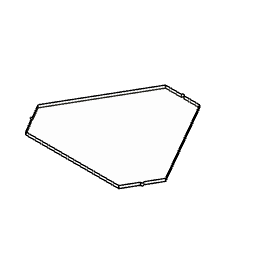
Zusammenbau v36 (Autodesk Fusion 360 archive; units mm, degrees)
design "Diffusor_Panel"
Autodesk Fusion 360 part; units mm, degrees
note: some values were not read from the file. Set by a fixed rule: the direction of a hole.
(part 1 of 2)
sketch "Skizze1" plane through (0, 0, 0) normal (0, 0, 1) x (1, 0, 0)
  line L0 (-53.4049, 0) -> (53.4049, 0)
  line L1 (53.4049, 0) -> (73.0348, 34)
  line L2 (73.0348, 34) -> (19.6299, 126.5)
  line L3 (19.6299, 126.5) -> (-19.6299, 126.5)
  line L4 (-19.6299, 126.5) -> (-73.0348, 34)
  line L5 (-73.0348, 34) -> (-53.4049, 0)
  line L6 (0, 0) -> (0, 126.5)
  line L7 (-63.2199, 17) -> (46.3324, 80.25)
  line L8 (63.2199, 17) -> (-46.3324, 80.25)
  circle A0 centre (0, 126.5) radius 1.4
  circle A1 centre (-63.2199, 17) radius 1.4
  circle A2 centre (63.2199, 17) radius 1.4
  point P0 (0, 53.5)
  dimension "d1" = 53.5
  dimension "d2" = 73
  dimension "d3" = 39.2598
  dimension "d4" = 106.8098
  dimension "d11" = 2.8
  dimension "d13" = 360
  constraint horizontal L0
  constraint parallel L0 L3
  constraint parallel L1 L4
  constraint equal L1 L3
  constraint equal L1 L5
  constraint equal L2 L4
  constraint equal L0 L2
  constraint coincident L6.start L0
  constraint coincident L6.start origin
  constraint coincident L3 L6.end
  constraint perpendicular L3 L6
  constraint symmetric L2 L4 L6
  constraint symmetric L1 L5 L6
  constraint midpoint L5 L7.start
  constraint midpoint L2 L7.end
  constraint midpoint L1 L8.start
  constraint midpoint L4 L8.end
  constraint coincident L7 P0
  constraint coincident L6 P0
  constraint coincident L6.end A0.centre
  measures "d1" distance of L0 P0
  measures "d2" distance of L3 P0
  measures "d3" distance of L2.end L3.end
  measures "d4" distance of L0.start L0.end
  measures "d11" diameter of A0
extrude "Extrusion1" add sketch "Skizze1" along normal blind 3
sketch "Skizze2" plane through (0, 0, 3) normal (0, 0, 1) x (-1, 0, 0)
  arc A0 (-62.5199, -15.7876) -> (-63.9199, -18.2124) centre (-63.2199, -17) ccw
  line L0 (-63.9199, -18.2124) -> (-73.0348, -34)
  line L1 (-73.0348, -34) -> (-19.6299, -126.5)
  line L2 (-19.6299, -126.5) -> (-1.4, -126.5)
  arc A1 (-1.4, -126.5) -> (1.4, -126.5) centre (0, -126.5) ccw
  line L3 (1.4, -126.5) -> (19.6299, -126.5)
  line L4 (19.6299, -126.5) -> (73.0348, -34)
  line L5 (73.0348, -34) -> (63.9199, -18.2124)
  arc A2 (63.9199, -18.2124) -> (62.5199, -15.7876) centre (63.2199, -17) ccw
  line L6 (62.5199, -15.7876) -> (53.4049, 0)
  line L7 (53.4049, 0) -> (-53.4049, 0)
  line L8 (-53.4049, 0) -> (-62.5199, -15.7876)
equation "d6 = 0deg 0'"
equation "d10 = 0deg 0'"
equation "d13 = 360deg 0'"

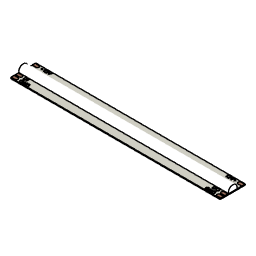
design "FCOB"
Autodesk Fusion 360 part; units mm, degrees
sketch "Skizze1" plane through (0, 0, 0) normal (1, 0, 0) x (0, 1, 0)
  line L0 (0, 0) -> (12, 0)
  line L1 (12, 0) -> (12, 0.4)
  line L2 (12, 0.4) -> (0, 0.4)
  line L3 (0, 0.4) -> (0, 0)
  arc A0 (8, 0.4) -> (4, 0.4) centre (6, 1.0093) ccw
  line L4 (6, 0.4) -> (6, 0)
  point P0 (6, 3.1)
  dimension "d1" = 0.4
  dimension "d2" = 12
  dimension "d3" = 3.1
  dimension "d4" = 4
  constraint horizontal L0
  constraint vertical L1
  constraint horizontal L2
  constraint vertical L3
  constraint coincident L0.start L3.end
  constraint coincident L2 A0.start
  constraint coincident L2 A0.end
  constraint midpoint L2 L4.start
  constraint midpoint L0 L4.end
  constraint coincident A0.centre L4
  constraint midpoint A0 P0
  measures "d1" distance of L0.start L2.end
  measures "d2" distance of L1.end L2.end
  measures "d3" distance of L0 P0
  measures "d4" distance of A0.end A0.start
extrude "Extrusion1" add sketch "Skizze1" along normal blind 100 contours L0 L2 L3 L4 | L0 L1 L2 L4 makes body 1
extrude "Extrusion2" add sketch "Skizze1" along normal up to surface (100 mm away) separate body contours L2 A0 makes body 2
sketch "Skizze2" plane through (0, 0, 0.4) normal (0, 0, 1) x (-1, 0, 0)
  line L0 (0, -12) -> (0, 0)
  line L1 (0, 0) -> (-100, 0)
  line L2 (-100, 0) -> (-100, -12)
  line L3 (-100, -12) -> (0, -12)
  line L4 (0, -0.25) -> (0, -1.75)
  line L5 (-1.75, -1.75) -> (0, -1.75)
  line L6 (0, -0.25) -> (-1.75, -0.25)
  arc A0 (-1.75, -0.25) -> (-1.75, -1.75) centre (-1.75, -1) ccw
  line L7 (0, -1) -> (-2.5, -1) construction
  dimension "d11" = 1.5
  dimension "d13" = 2.5
  dimension "d14" = 0.25
  constraint coincident L0 L4.start
  constraint coincident L0 L4.end
  constraint perpendicular L4 L5
  constraint perpendicular L4 L6
  constraint tangent L6 A0
  constraint tangent L5 A0
  constraint midpoint L4 L7.start
  constraint midpoint A0 L7.end
  measures "d11" distance of L4.start L4.end
  measures "d13" distance of L7.start L7.end
  measures "d14" distance of L1 L6
extrude "Extrusion3" add sketch "Skizze2" along normal blind 0.035 contours L0 L4 L5 L6 A0 bodies 1
pattern_linear "R-Anordnung1" count 2 spacing 2 along (0, 1, 0) of "Extrusion3"
pattern_linear "R-Anordnung2" count 2 spacing 10 along (0, 1, 0) of "Extrusion3"
ref_plane "Arbeitsebene1" through (50, 6, 0.2175) normal (-1, 0, 0) x (0, -1, 0)
mirror "Spiegeln1" about plane through (50, 6, 0.2175) normal (-1, 0, 0) of "Extrusion3", "R-Anordnung1", "R-Anordnung2"
sketch "Skizze3" plane through (0, 0, 0.4) normal (0, 0, 1) x (-1, 0, 0)
  line L0 (-100, -10.25) -> (-98.25, -10.25)
  arc A0 (-98.25, -11.75) -> (-98.25, -10.25) centre (-98.25, -11) ccw
  line L1 (-98.25, -11.75) -> (-100, -11.75)
  line L2 (-100, -11.75) -> (-100, -12)
  line L3 (-100, -12) -> (0, -12)
  line L4 (0, -12) -> (0, -11.75)
  line L5 (0, -11.75) -> (-1.75, -11.75)
  arc A1 (-1.75, -10.25) -> (-1.75, -11.75) centre (-1.75, -11) ccw
  line L6 (-1.75, -10.25) -> (0, -10.25)
  line L7 (0, -10.25) -> (0, -3.75)
  line L8 (0, -3.75) -> (-1.75, -3.75)
  arc A2 (-1.75, -2.25) -> (-1.75, -3.75) centre (-1.75, -3) ccw
  line L9 (-1.75, -2.25) -> (0, -2.25)
  line L10 (0, -2.25) -> (0, -1.75)
  line L11 (0, -1.75) -> (-1.75, -1.75)
  arc A3 (-1.75, -0.25) -> (-1.75, -1.75) centre (-1.75, -1) ccw
  line L12 (-1.75, -0.25) -> (0, -0.25)
  line L13 (0, -0.25) -> (0, 0)
  line L14 (0, 0) -> (-100, 0)
  line L15 (-100, 0) -> (-100, -0.25)
  line L16 (-100, -0.25) -> (-98.25, -0.25)
  arc A4 (-98.25, -1.75) -> (-98.25, -0.25) centre (-98.25, -1) ccw
  line L17 (-98.25, -1.75) -> (-100, -1.75)
  line L18 (-100, -1.75) -> (-100, -2.25)
  line L19 (-100, -2.25) -> (-98.25, -2.25)
  arc A5 (-98.25, -3.75) -> (-98.25, -2.25) centre (-98.25, -3) ccw
  line L20 (-98.25, -3.75) -> (-100, -3.75)
  line L21 (-100, -3.75) -> (-100, -10.25)
  line L22 (-4.252, -0.8383) -> (-4.252, -1.0143)
  line L23 (-4.252, -1.0143) -> (-4.8874, -1.0153)
  line L24 (-4.8874, -1.0153) -> (-4.8874, -0.4587)
  spline S0 degree 2 poles (-4.8874, -0.4587) (-4.7411, -0.3421) (-4.5856, -0.2833) knots 0 0 0 1 1 1
  spline S1 degree 2 poles (-4.5856, -0.2833) (-4.4301, -0.2244) (-4.2664, -0.2244) knots 0 0 0 1 1 1
  spline S2 degree 2 poles (-4.2664, -0.2244) (-4.0454, -0.2244) (-3.8648, -0.3191) knots 0 0 0 1 1 1
  spline S3 degree 2 poles (-3.8648, -0.3191) (-3.6842, -0.4137) (-3.5921, -0.5928) knots 0 0 0 1 1 1
  spline S4 degree 2 poles (-3.5921, -0.5928) (-3.5, -0.7718) (-3.5, -0.9928) knots 0 0 0 1 1 1
  spline S5 degree 2 poles (-3.5, -0.9928) (-3.5, -1.2118) (-3.5916, -1.4016) knots 0 0 0 1 1 1
  spline S6 degree 2 poles (-3.5916, -1.4016) (-3.6832, -1.5914) (-3.855, -1.6835) knots 0 0 0 1 1 1
  spline S7 degree 2 poles (-3.855, -1.6835) (-4.0269, -1.7756) (-4.251, -1.7756) knots 0 0 0 1 1 1
  spline S8 degree 2 poles (-4.251, -1.7756) (-4.4137, -1.7756) (-4.5452, -1.7229) knots 0 0 0 1 1 1
  spline S9 degree 2 poles (-4.5452, -1.7229) (-4.6767, -1.6702) (-4.7514, -1.5761) knots 0 0 0 1 1 1
  spline S10 degree 2 poles (-4.7514, -1.5761) (-4.8261, -1.4819) (-4.8649, -1.3305) knots 0 0 0 1 1 1
  line L25 (-4.8649, -1.3305) -> (-4.6859, -1.2814)
  spline S11 degree 2 poles (-4.6859, -1.2814) (-4.6521, -1.396) (-4.602, -1.4615) knots 0 0 0 1 1 1
  spline S12 degree 2 poles (-4.602, -1.4615) (-4.5518, -1.5269) (-4.4587, -1.5663) knots 0 0 0 1 1 1
  spline S13 degree 2 poles (-4.4587, -1.5663) (-4.3656, -1.6057) (-4.252, -1.6057) knots 0 0 0 1 1 1
  spline S14 degree 2 poles (-4.252, -1.6057) (-4.116, -1.6057) (-4.0167, -1.5643) knots 0 0 0 1 1 1
  spline S15 degree 2 poles (-4.0167, -1.5643) (-3.9175, -1.5229) (-3.8566, -1.4553) knots 0 0 0 1 1 1
  spline S16 degree 2 poles (-3.8566, -1.4553) (-3.7957, -1.3878) (-3.7619, -1.307) knots 0 0 0 1 1 1
  spline S17 degree 2 poles (-3.7619, -1.307) (-3.7046, -1.1678) (-3.7046, -1.0051) knots 0 0 0 1 1 1
  spline S18 degree 2 poles (-3.7046, -1.0051) (-3.7046, -0.8046) (-3.7737, -0.6695) knots 0 0 0 1 1 1
  spline S19 degree 2 poles (-3.7737, -0.6695) (-3.8428, -0.5344) (-3.9748, -0.469) knots 0 0 0 1 1 1
  spline S20 degree 2 poles (-3.9748, -0.469) (-4.1068, -0.4035) (-4.2551, -0.4035) knots 0 0 0 1 1 1
  spline S21 degree 2 poles (-4.2551, -0.4035) (-4.384, -0.4035) (-4.5068, -0.4531) knots 0 0 0 1 1 1
  spline S22 degree 2 poles (-4.5068, -0.4531) (-4.6296, -0.5027) (-4.693, -0.559) knots 0 0 0 1 1 1
  line L26 (-4.693, -0.559) -> (-4.693, -0.8383)
  line L27 (-4.693, -0.8383) -> (-4.252, -0.8383)
  line L28 (-5.178, -0.25) -> (-5.178, -1.75)
  line L29 (-5.178, -1.75) -> (-5.3817, -1.75)
  line L30 (-5.3817, -1.75) -> (-6.1695, -0.5723)
  line L31 (-6.1695, -0.5723) -> (-6.1695, -1.75)
  line L32 (-6.1695, -1.75) -> (-6.3598, -1.75)
  line L33 (-6.3598, -1.75) -> (-6.3598, -0.25)
  line L34 (-6.3598, -0.25) -> (-6.1562, -0.25)
  line L35 (-6.1562, -0.25) -> (-5.3683, -1.4287)
  line L36 (-5.3683, -1.4287) -> (-5.3683, -0.25)
  line L37 (-5.3683, -0.25) -> (-5.178, -0.25)
  line L38 (-6.6934, -0.25) -> (-6.6934, -1.75)
  line L39 (-6.6934, -1.75) -> (-7.2101, -1.75)
  spline S23 degree 2 poles (-7.2101, -1.75) (-7.3851, -1.75) (-7.4771, -1.7285) knots 0 0 0 1 1 1
  spline S24 degree 2 poles (-7.4771, -1.7285) (-7.6061, -1.6988) (-7.6971, -1.6211) knots 0 0 0 1 1 1
  spline S25 degree 2 poles (-7.6971, -1.6211) (-7.8158, -1.5208) (-7.8747, -1.3648) knots 0 0 0 1 1 1
  spline S26 degree 2 poles (-7.8747, -1.3648) (-7.9335, -1.2087) (-7.9335, -1.0082) knots 0 0 0 1 1 1
  spline S27 degree 2 poles (-7.9335, -1.0082) (-7.9335, -0.8373) (-7.8936, -0.7053) knots 0 0 0 1 1 1
  spline S28 degree 2 poles (-7.8936, -0.7053) (-7.8537, -0.5733) (-7.7913, -0.4869) knots 0 0 0 1 1 1
  spline S29 degree 2 poles (-7.7913, -0.4869) (-7.7289, -0.4004) (-7.6547, -0.3508) knots 0 0 0 1 1 1
  spline S30 degree 2 poles (-7.6547, -0.3508) (-7.5805, -0.3012) (-7.4756, -0.2756) knots 0 0 0 1 1 1
  spline S31 degree 2 poles (-7.4756, -0.2756) (-7.3707, -0.25) (-7.2347, -0.25) knots 0 0 0 1 1 1
  line L40 (-7.2347, -0.25) -> (-6.6934, -0.25)
  line L41 (-6.8919, -0.427) -> (-7.2121, -0.427)
  spline S32 degree 2 poles (-7.2121, -0.427) (-7.3605, -0.427) (-7.4449, -0.4546) knots 0 0 0 1 1 1
  spline S33 degree 2 poles (-7.4449, -0.4546) (-7.5293, -0.4823) (-7.5795, -0.5324) knots 0 0 0 1 1 1
  spline S34 degree 2 poles (-7.5795, -0.5324) (-7.6501, -0.603) (-7.6895, -0.7222) knots 0 0 0 1 1 1
  spline S35 degree 2 poles (-7.6895, -0.7222) (-7.7289, -0.8414) (-7.7289, -1.0113) knots 0 0 0 1 1 1
  spline S36 degree 2 poles (-7.7289, -1.0113) (-7.7289, -1.2466) (-7.6516, -1.373) knots 0 0 0 1 1 1
  spline S37 degree 2 poles (-7.6516, -1.373) (-7.5744, -1.4993) (-7.4638, -1.5423) knots 0 0 0 1 1 1
  spline S38 degree 2 poles (-7.4638, -1.5423) (-7.384, -1.573) (-7.207, -1.573) knots 0 0 0 1 1 1
  line L42 (-7.207, -1.573) -> (-6.8919, -1.573)
  line L43 (-6.8919, -1.573) -> (-6.8919, -0.427)
  line L44 (-3.5, -2.25) -> (-3.5, -3.75)
  line L45 (-3.5, -3.75) -> (-4.0167, -3.75)
  spline S39 degree 2 poles (-4.0167, -3.75) (-4.1917, -3.75) (-4.2838, -3.7285) knots 0 0 0 1 1 1
  spline S40 degree 2 poles (-4.2838, -3.7285) (-4.4127, -3.6988) (-4.5038, -3.6211) knots 0 0 0 1 1 1
  spline S41 degree 2 poles (-4.5038, -3.6211) (-4.6224, -3.5208) (-4.6813, -3.3648) knots 0 0 0 1 1 1
  spline S42 degree 2 poles (-4.6813, -3.3648) (-4.7401, -3.2087) (-4.7401, -3.0082) knots 0 0 0 1 1 1
  spline S43 degree 2 poles (-4.7401, -3.0082) (-4.7401, -2.8373) (-4.7002, -2.7053) knots 0 0 0 1 1 1
  spline S44 degree 2 poles (-4.7002, -2.7053) (-4.6603, -2.5733) (-4.5979, -2.4869) knots 0 0 0 1 1 1
  spline S45 degree 2 poles (-4.5979, -2.4869) (-4.5355, -2.4004) (-4.4613, -2.3508) knots 0 0 0 1 1 1
  spline S46 degree 2 poles (-4.4613, -2.3508) (-4.3871, -2.3012) (-4.2822, -2.2756) knots 0 0 0 1 1 1
  spline S47 degree 2 poles (-4.2822, -2.2756) (-4.1774, -2.25) (-4.0413, -2.25) knots 0 0 0 1 1 1
  line L46 (-4.0413, -2.25) -> (-3.5, -2.25)
  line L47 (-3.6985, -2.427) -> (-4.0188, -2.427)
  spline S48 degree 2 poles (-4.0188, -2.427) (-4.1671, -2.427) (-4.2515, -2.4546) knots 0 0 0 1 1 1
  spline S49 degree 2 poles (-4.2515, -2.4546) (-4.3359, -2.4823) (-4.3861, -2.5324) knots 0 0 0 1 1 1
  spline S50 degree 2 poles (-4.3861, -2.5324) (-4.4567, -2.603) (-4.4961, -2.7222) knots 0 0 0 1 1 1
  spline S51 degree 2 poles (-4.4961, -2.7222) (-4.5355, -2.8414) (-4.5355, -3.0113) knots 0 0 0 1 1 1
  spline S52 degree 2 poles (-4.5355, -3.0113) (-4.5355, -3.2466) (-4.4582, -3.373) knots 0 0 0 1 1 1
  spline S53 degree 2 poles (-4.4582, -3.373) (-4.381, -3.4993) (-4.2705, -3.5423) knots 0 0 0 1 1 1
  spline S54 degree 2 poles (-4.2705, -3.5423) (-4.1907, -3.573) (-4.0136, -3.573) knots 0 0 0 1 1 1
  line L48 (-4.0136, -3.573) -> (-3.6985, -3.573)
  line L49 (-3.6985, -3.573) -> (-3.6985, -2.427)
  line L50 (-5.0471, -2.25) -> (-5.0471, -3.75)
  line L51 (-5.0471, -3.75) -> (-5.2456, -3.75)
  line L52 (-5.2456, -3.75) -> (-5.2456, -2.25)
  line L53 (-5.2456, -2.25) -> (-5.0471, -2.25)
  line L54 (-3.9083, -10.4925) -> (-3.9083, -10.9038)
  line L55 (-3.9083, -10.9038) -> (-3.5, -10.9038)
  line L56 (-3.5, -10.9038) -> (-3.5, -11.0757)
  line L57 (-3.5, -11.0757) -> (-3.9083, -11.0757)
  line L58 (-3.9083, -11.0757) -> (-3.9083, -11.484)
  line L59 (-3.9083, -11.484) -> (-4.0822, -11.484)
  line L60 (-4.0822, -11.484) -> (-4.0822, -11.0757)
  line L61 (-4.0822, -11.0757) -> (-4.4905, -11.0757)
  line L62 (-4.4905, -11.0757) -> (-4.4905, -10.9038)
  line L63 (-4.4905, -10.9038) -> (-4.0822, -10.9038)
  line L64 (-4.0822, -10.9038) -> (-4.0822, -10.4925)
  line L65 (-4.0822, -10.4925) -> (-3.9083, -10.4925)
  line L66 (-5.3878, -10.25) -> (-5.2036, -10.25)
  line L67 (-5.2036, -10.25) -> (-5.2036, -11.4236)
  spline S55 degree 2 poles (-5.2036, -11.4236) (-5.1371, -11.3602) (-5.0292, -11.2967) knots 0 0 0 1 1 1
  spline S56 degree 2 poles (-5.0292, -11.2967) (-4.9212, -11.2333) (-4.8353, -11.2016) knots 0 0 0 1 1 1
  line L68 (-4.8353, -11.2016) -> (-4.8353, -11.3796)
  spline S57 degree 2 poles (-4.8353, -11.3796) (-4.9898, -11.4523) (-5.1054, -11.5556) knots 0 0 0 1 1 1
  spline S58 degree 2 poles (-5.1054, -11.5556) (-5.221, -11.6589) (-5.2691, -11.7561) knots 0 0 0 1 1 1
  line L69 (-5.2691, -11.7561) -> (-5.3878, -11.7561)
  line L70 (-5.3878, -11.7561) -> (-5.3878, -10.25)
  line L71 (-6.8274, -10.427) -> (-6.8274, -10.25)
  line L72 (-6.8274, -10.25) -> (-5.8359, -10.25)
  spline S59 degree 2 poles (-5.8359, -10.25) (-5.8339, -10.3165) (-5.8574, -10.3779) knots 0 0 0 1 1 1
  spline S60 degree 2 poles (-5.8574, -10.3779) (-5.8953, -10.4792) (-5.9787, -10.5774) knots 0 0 0 1 1 1
  spline S61 degree 2 poles (-5.9787, -10.5774) (-6.0621, -10.6756) (-6.2196, -10.8046) knots 0 0 0 1 1 1
  spline S62 degree 2 poles (-6.2196, -10.8046) (-6.4642, -11.0051) (-6.5501, -11.1223) knots 0 0 0 1 1 1
  spline S63 degree 2 poles (-6.5501, -11.1223) (-6.6361, -11.2394) (-6.6361, -11.3438) knots 0 0 0 1 1 1
  spline S64 degree 2 poles (-6.6361, -11.3438) (-6.6361, -11.4533) (-6.5578, -11.5285) knots 0 0 0 1 1 1
  spline S65 degree 2 poles (-6.5578, -11.5285) (-6.4795, -11.6037) (-6.3537, -11.6037) knots 0 0 0 1 1 1
  spline S66 degree 2 poles (-6.3537, -11.6037) (-6.2207, -11.6037) (-6.1409, -11.5239) knots 0 0 0 1 1 1
  spline S67 degree 2 poles (-6.1409, -11.5239) (-6.0611, -11.4441) (-6.06, -11.3029) knots 0 0 0 1 1 1
  line L73 (-6.06, -11.3029) -> (-5.8707, -11.3223)
  spline S68 degree 2 poles (-5.8707, -11.3223) (-5.8902, -11.5341) (-6.0171, -11.6451) knots 0 0 0 1 1 1
  spline S69 degree 2 poles (-6.0171, -11.6451) (-6.1439, -11.7561) (-6.3578, -11.7561) knots 0 0 0 1 1 1
  spline S70 degree 2 poles (-6.3578, -11.7561) (-6.5737, -11.7561) (-6.6995, -11.6364) knots 0 0 0 1 1 1
  spline S71 degree 2 poles (-6.6995, -11.6364) (-6.8254, -11.5167) (-6.8254, -11.3397) knots 0 0 0 1 1 1
  spline S72 degree 2 poles (-6.8254, -11.3397) (-6.8254, -11.2497) (-6.7885, -11.1627) knots 0 0 0 1 1 1
  spline S73 degree 2 poles (-6.7885, -11.1627) (-6.7517, -11.0757) (-6.6663, -10.9795) knots 0 0 0 1 1 1
  spline S74 degree 2 poles (-6.6663, -10.9795) (-6.5808, -10.8834) (-6.3823, -10.7156) knots 0 0 0 1 1 1
  spline S75 degree 2 poles (-6.3823, -10.7156) (-6.2166, -10.5764) (-6.1695, -10.5268) knots 0 0 0 1 1 1
  spline S76 degree 2 poles (-6.1695, -10.5268) (-6.1224, -10.4771) (-6.0917, -10.427) knots 0 0 0 1 1 1
  line L74 (-6.0917, -10.427) -> (-6.8274, -10.427)
  line L75 (-7.5283, -10.25) -> (-6.9471, -11.75)
  line L76 (-6.9471, -11.75) -> (-7.162, -11.75)
  line L77 (-7.162, -11.75) -> (-7.5518, -10.6603)
  spline S77 degree 2 poles (-7.5518, -10.6603) (-7.5989, -10.5293) (-7.6306, -10.4147) knots 0 0 0 1 1 1
  spline S78 degree 2 poles (-7.6306, -10.4147) (-7.6654, -10.5375) (-7.7115, -10.6603) knots 0 0 0 1 1 1
  line L78 (-7.7115, -10.6603) -> (-8.1166, -11.75)
  line L79 (-8.1166, -11.75) -> (-8.3192, -11.75)
  line L80 (-8.3192, -11.75) -> (-7.7319, -10.25)
  line L81 (-7.7319, -10.25) -> (-7.5283, -10.25)
extrude "Extrusion4" add sketch "Skizze3" along normal blind 0.01 contours L22 L23 L24 S0 S1 S2 S3 S4 S5 S6 S7 S8 S9 S10 L25 S11 S12 S13 S14 S15 S16 S17 S18 S19 S20 S21 S22 L26 L27 | L28 L29 L30 L31 L32 L33 L34 L35 L36 L37 | L38 L39 S23 S24 S25 S26 S27 S28 S29 S30 S31 L40 | L44 L45 S39 S40 S41 S42 S43 S44 S45 S46 S47 L46 | L50 L51 L52 L53 | L54 L55 L56 L57 L58 L59 L60 L61 L62 L63 L64 L65 | L66 L67 S55 S56 L68 S57 S58 L69 L70 | L71 L72 S59 S60 S61 S62 S63 S64 S65 S66 S67 L73 S68 S69 S70 S71 S72 S73 S74 S75 S76 L74 | L75 L76 L77 S77 S78 L78 L79 L80 L81 bodies 1
sketch "Skizze4" plane through (0, 0, 0.4) normal (0, 0, 1) x (-1, 0, 0)
  line L0 (-7.7319, -10.25) -> (-7.5283, -10.25)
  line L1 (-7.5283, -10.25) -> (-6.9471, -11.75)
  line L2 (-6.9471, -11.75) -> (-7.162, -11.75)
  line L3 (-7.162, -11.75) -> (-7.5518, -10.6603)
  spline S0 degree 2 poles (-7.5518, -10.6603) (-7.5989, -10.5293) (-7.6306, -10.4147) knots 0 0 0 1 1 1
  spline S1 degree 2 poles (-7.6306, -10.4147) (-7.6654, -10.5375) (-7.7115, -10.6603) knots 0 0 0 1 1 1
  line L4 (-7.7115, -10.6603) -> (-8.1166, -11.75)
  line L5 (-8.1166, -11.75) -> (-8.3192, -11.75)
  line L6 (-8.3192, -11.75) -> (-7.7319, -10.25)
  line L7 (-5.2456, -2.25) -> (-5.0471, -2.25)
  line L8 (-5.0471, -2.25) -> (-5.0471, -3.75)
  line L9 (-5.0471, -3.75) -> (-5.2456, -3.75)
  line L10 (-5.2456, -3.75) -> (-5.2456, -2.25)
  line L11 (-4.693, -0.8383) -> (-4.252, -0.8383)
  line L12 (-4.252, -0.8383) -> (-4.252, -1.0143)
  line L13 (-4.252, -1.0143) -> (-4.8874, -1.0153)
  line L14 (-4.8874, -1.0153) -> (-4.8874, -0.4587)
  spline S2 degree 2 poles (-4.8874, -0.4587) (-4.7411, -0.3421) (-4.5856, -0.2833) knots 0 0 0 1 1 1
  spline S3 degree 2 poles (-4.5856, -0.2833) (-4.4301, -0.2244) (-4.2664, -0.2244) knots 0 0 0 1 1 1
  spline S4 degree 2 poles (-4.2664, -0.2244) (-4.0454, -0.2244) (-3.8648, -0.3191) knots 0 0 0 1 1 1
  spline S5 degree 2 poles (-3.8648, -0.3191) (-3.6842, -0.4137) (-3.5921, -0.5928) knots 0 0 0 1 1 1
  spline S6 degree 2 poles (-3.5921, -0.5928) (-3.5, -0.7718) (-3.5, -0.9928) knots 0 0 0 1 1 1
  spline S7 degree 2 poles (-3.5, -0.9928) (-3.5, -1.2118) (-3.5916, -1.4016) knots 0 0 0 1 1 1
  spline S8 degree 2 poles (-3.5916, -1.4016) (-3.6832, -1.5914) (-3.855, -1.6835) knots 0 0 0 1 1 1
  spline S9 degree 2 poles (-3.855, -1.6835) (-4.0269, -1.7756) (-4.251, -1.7756) knots 0 0 0 1 1 1
  spline S10 degree 2 poles (-4.251, -1.7756) (-4.4137, -1.7756) (-4.5452, -1.7229) knots 0 0 0 1 1 1
  spline S11 degree 2 poles (-4.5452, -1.7229) (-4.6767, -1.6702) (-4.7514, -1.5761) knots 0 0 0 1 1 1
  spline S12 degree 2 poles (-4.7514, -1.5761) (-4.8261, -1.4819) (-4.8649, -1.3305) knots 0 0 0 1 1 1
  line L15 (-4.8649, -1.3305) -> (-4.6859, -1.2814)
  spline S13 degree 2 poles (-4.6859, -1.2814) (-4.6521, -1.396) (-4.602, -1.4615) knots 0 0 0 1 1 1
  spline S14 degree 2 poles (-4.602, -1.4615) (-4.5518, -1.5269) (-4.4587, -1.5663) knots 0 0 0 1 1 1
  spline S15 degree 2 poles (-4.4587, -1.5663) (-4.3656, -1.6057) (-4.252, -1.6057) knots 0 0 0 1 1 1
  spline S16 degree 2 poles (-4.252, -1.6057) (-4.116, -1.6057) (-4.0167, -1.5643) knots 0 0 0 1 1 1
  spline S17 degree 2 poles (-4.0167, -1.5643) (-3.9175, -1.5229) (-3.8566, -1.4553) knots 0 0 0 1 1 1
  spline S18 degree 2 poles (-3.8566, -1.4553) (-3.7957, -1.3878) (-3.7619, -1.307) knots 0 0 0 1 1 1
  spline S19 degree 2 poles (-3.7619, -1.307) (-3.7046, -1.1678) (-3.7046, -1.0051) knots 0 0 0 1 1 1
  spline S20 degree 2 poles (-3.7046, -1.0051) (-3.7046, -0.8046) (-3.7737, -0.6695) knots 0 0 0 1 1 1
  spline S21 degree 2 poles (-3.7737, -0.6695) (-3.8428, -0.5344) (-3.9748, -0.469) knots 0 0 0 1 1 1
  spline S22 degree 2 poles (-3.9748, -0.469) (-4.1068, -0.4035) (-4.2551, -0.4035) knots 0 0 0 1 1 1
  spline S23 degree 2 poles (-4.2551, -0.4035) (-4.384, -0.4035) (-4.5068, -0.4531) knots 0 0 0 1 1 1
  spline S24 degree 2 poles (-4.5068, -0.4531) (-4.6296, -0.5027) (-4.693, -0.559) knots 0 0 0 1 1 1
  line L16 (-4.693, -0.559) -> (-4.693, -0.8383)
  line L17 (-7.2347, -0.25) -> (-6.6934, -0.25)
  line L18 (-6.6934, -0.25) -> (-6.6934, -1.75)
  line L19 (-6.6934, -1.75) -> (-7.2101, -1.75)
  spline S25 degree 2 poles (-7.2101, -1.75) (-7.3851, -1.75) (-7.4771, -1.7285) knots 0 0 0 1 1 1
  spline S26 degree 2 poles (-7.4771, -1.7285) (-7.6061, -1.6988) (-7.6971, -1.6211) knots 0 0 0 1 1 1
  spline S27 degree 2 poles (-7.6971, -1.6211) (-7.8158, -1.5208) (-7.8747, -1.3648) knots 0 0 0 1 1 1
  spline S28 degree 2 poles (-7.8747, -1.3648) (-7.9335, -1.2087) (-7.9335, -1.0082) knots 0 0 0 1 1 1
  spline S29 degree 2 poles (-7.9335, -1.0082) (-7.9335, -0.8373) (-7.8936, -0.7053) knots 0 0 0 1 1 1
  spline S30 degree 2 poles (-7.8936, -0.7053) (-7.8537, -0.5733) (-7.7913, -0.4869) knots 0 0 0 1 1 1
  spline S31 degree 2 poles (-7.7913, -0.4869) (-7.7289, -0.4004) (-7.6547, -0.3508) knots 0 0 0 1 1 1
  spline S32 degree 2 poles (-7.6547, -0.3508) (-7.5805, -0.3012) (-7.4756, -0.2756) knots 0 0 0 1 1 1
  spline S33 degree 2 poles (-7.4756, -0.2756) (-7.3707, -0.25) (-7.2347, -0.25) knots 0 0 0 1 1 1
  line L20 (-5.3878, -11.7561) -> (-5.3878, -10.25)
  line L21 (-5.3878, -10.25) -> (-5.2036, -10.25)
  line L22 (-5.2036, -10.25) -> (-5.2036, -11.4236)
  spline S34 degree 2 poles (-5.2036, -11.4236) (-5.1371, -11.3602) (-5.0292, -11.2967) knots 0 0 0 1 1 1
  spline S35 degree 2 poles (-5.0292, -11.2967) (-4.9212, -11.2333) (-4.8353, -11.2016) knots 0 0 0 1 1 1
  line L23 (-4.8353, -11.2016) -> (-4.8353, -11.3796)
  spline S36 degree 2 poles (-4.8353, -11.3796) (-4.9898, -11.4523) (-5.1054, -11.5556) knots 0 0 0 1 1 1
  spline S37 degree 2 poles (-5.1054, -11.5556) (-5.221, -11.6589) (-5.2691, -11.7561) knots 0 0 0 1 1 1
  line L24 (-5.2691, -11.7561) -> (-5.3878, -11.7561)
  line L25 (-100, -10.25) -> (-98.25, -10.25)
  arc A0 (-98.25, -11.75) -> (-98.25, -10.25) centre (-98.25, -11) ccw
  line L26 (-98.25, -11.75) -> (-100, -11.75)
  line L27 (-100, -11.75) -> (-100, -12)
  line L28 (-100, -12) -> (0, -12)
  line L29 (0, -12) -> (0, -11.75)
  line L30 (0, -11.75) -> (-1.75, -11.75)
  arc A1 (-1.75, -10.25) -> (-1.75, -11.75) centre (-1.75, -11) ccw
  line L31 (-1.75, -10.25) -> (0, -10.25)
  line L32 (0, -10.25) -> (0, -3.75)
  line L33 (0, -3.75) -> (-1.75, -3.75)
  arc A2 (-1.75, -2.25) -> (-1.75, -3.75) centre (-1.75, -3) ccw
  line L34 (-1.75, -2.25) -> (0, -2.25)
  line L35 (0, -2.25) -> (0, -1.75)
  line L36 (0, -1.75) -> (-1.75, -1.75)
  arc A3 (-1.75, -0.25) -> (-1.75, -1.75) centre (-1.75, -1) ccw
  line L37 (-1.75, -0.25) -> (0, -0.25)
  line L38 (0, -0.25) -> (0, 0)
  line L39 (0, 0) -> (-100, 0)
  line L40 (-100, 0) -> (-100, -0.25)
  line L41 (-100, -0.25) -> (-98.25, -0.25)
  arc A4 (-98.25, -1.75) -> (-98.25, -0.25) centre (-98.25, -1) ccw
  line L42 (-98.25, -1.75) -> (-100, -1.75)
  line L43 (-100, -1.75) -> (-100, -2.25)
  line L44 (-100, -2.25) -> (-98.25, -2.25)
  arc A5 (-98.25, -3.75) -> (-98.25, -2.25) centre (-98.25, -3) ccw
  line L45 (-98.25, -3.75) -> (-100, -3.75)
  line L46 (-100, -3.75) -> (-100, -10.25)
  line L47 (-5.3683, -0.25) -> (-5.178, -0.25)
  line L48 (-5.178, -0.25) -> (-5.178, -1.75)
  line L49 (-5.178, -1.75) -> (-5.3817, -1.75)
  line L50 (-5.3817, -1.75) -> (-6.1695, -0.5723)
  line L51 (-6.1695, -0.5723) -> (-6.1695, -1.75)
  line L52 (-6.1695, -1.75) -> (-6.3598, -1.75)
  line L53 (-6.3598, -1.75) -> (-6.3598, -0.25)
  line L54 (-6.3598, -0.25) -> (-6.1562, -0.25)
  line L55 (-6.1562, -0.25) -> (-5.3683, -1.4287)
  line L56 (-5.3683, -1.4287) -> (-5.3683, -0.25)
  line L57 (-4.0822, -10.4925) -> (-3.9083, -10.4925)
  line L58 (-3.9083, -10.4925) -> (-3.9083, -10.9038)
  line L59 (-3.9083, -10.9038) -> (-3.5, -10.9038)
  line L60 (-3.5, -10.9038) -> (-3.5, -11.0757)
  line L61 (-3.5, -11.0757) -> (-3.9083, -11.0757)
  line L62 (-3.9083, -11.0757) -> (-3.9083, -11.484)
  line L63 (-3.9083, -11.484) -> (-4.0822, -11.484)
  line L64 (-4.0822, -11.484) -> (-4.0822, -11.0757)
  line L65 (-4.0822, -11.0757) -> (-4.4905, -11.0757)
  line L66 (-4.4905, -11.0757) -> (-4.4905, -10.9038)
  line L67 (-4.4905, -10.9038) -> (-4.0822, -10.9038)
  line L68 (-4.0822, -10.9038) -> (-4.0822, -10.4925)
  line L69 (-6.0917, -10.427) -> (-6.8274, -10.427)
  line L70 (-6.8274, -10.427) -> (-6.8274, -10.25)
  line L71 (-6.8274, -10.25) -> (-5.8359, -10.25)
  spline S38 degree 2 poles (-5.8359, -10.25) (-5.8339, -10.3165) (-5.8574, -10.3779) knots 0 0 0 1 1 1
  spline S39 degree 2 poles (-5.8574, -10.3779) (-5.8953, -10.4792) (-5.9787, -10.5774) knots 0 0 0 1 1 1
  spline S40 degree 2 poles (-5.9787, -10.5774) (-6.0621, -10.6756) (-6.2196, -10.8046) knots 0 0 0 1 1 1
  spline S41 degree 2 poles (-6.2196, -10.8046) (-6.4642, -11.0051) (-6.5501, -11.1223) knots 0 0 0 1 1 1
  spline S42 degree 2 poles (-6.5501, -11.1223) (-6.6361, -11.2394) (-6.6361, -11.3438) knots 0 0 0 1 1 1
  spline S43 degree 2 poles (-6.6361, -11.3438) (-6.6361, -11.4533) (-6.5578, -11.5285) knots 0 0 0 1 1 1
  spline S44 degree 2 poles (-6.5578, -11.5285) (-6.4795, -11.6037) (-6.3537, -11.6037) knots 0 0 0 1 1 1
  spline S45 degree 2 poles (-6.3537, -11.6037) (-6.2207, -11.6037) (-6.1409, -11.5239) knots 0 0 0 1 1 1
  spline S46 degree 2 poles (-6.1409, -11.5239) (-6.0611, -11.4441) (-6.06, -11.3029) knots 0 0 0 1 1 1
  line L72 (-6.06, -11.3029) -> (-5.8707, -11.3223)
  spline S47 degree 2 poles (-5.8707, -11.3223) (-5.8902, -11.5341) (-6.0171, -11.6451) knots 0 0 0 1 1 1
  spline S48 degree 2 poles (-6.0171, -11.6451) (-6.1439, -11.7561) (-6.3578, -11.7561) knots 0 0 0 1 1 1
  spline S49 degree 2 poles (-6.3578, -11.7561) (-6.5737, -11.7561) (-6.6995, -11.6364) knots 0 0 0 1 1 1
  spline S50 degree 2 poles (-6.6995, -11.6364) (-6.8254, -11.5167) (-6.8254, -11.3397) knots 0 0 0 1 1 1
  spline S51 degree 2 poles (-6.8254, -11.3397) (-6.8254, -11.2497) (-6.7885, -11.1627) knots 0 0 0 1 1 1
  spline S52 degree 2 poles (-6.7885, -11.1627) (-6.7517, -11.0757) (-6.6663, -10.9795) knots 0 0 0 1 1 1
  spline S53 degree 2 poles (-6.6663, -10.9795) (-6.5808, -10.8834) (-6.3823, -10.7156) knots 0 0 0 1 1 1
  spline S54 degree 2 poles (-6.3823, -10.7156) (-6.2166, -10.5764) (-6.1695, -10.5268) knots 0 0 0 1 1 1
  spline S55 degree 2 poles (-6.1695, -10.5268) (-6.1224, -10.4771) (-6.0917, -10.427) knots 0 0 0 1 1 1
  line L73 (-4.0413, -2.25) -> (-3.5, -2.25)
  line L74 (-3.5, -2.25) -> (-3.5, -3.75)
  line L75 (-3.5, -3.75) -> (-4.0167, -3.75)
  spline S56 degree 2 poles (-4.0167, -3.75) (-4.1917, -3.75) (-4.2838, -3.7285) knots 0 0 0 1 1 1
  spline S57 degree 2 poles (-4.2838, -3.7285) (-4.4127, -3.6988) (-4.5038, -3.6211) knots 0 0 0 1 1 1
  spline S58 degree 2 poles (-4.5038, -3.6211) (-4.6224, -3.5208) (-4.6813, -3.3648) knots 0 0 0 1 1 1
  spline S59 degree 2 poles (-4.6813, -3.3648) (-4.7401, -3.2087) (-4.7401, -3.0082) knots 0 0 0 1 1 1
  spline S60 degree 2 poles (-4.7401, -3.0082) (-4.7401, -2.8373) (-4.7002, -2.7053) knots 0 0 0 1 1 1
  spline S61 degree 2 poles (-4.7002, -2.7053) (-4.6603, -2.5733) (-4.5979, -2.4869) knots 0 0 0 1 1 1
  spline S62 degree 2 poles (-4.5979, -2.4869) (-4.5355, -2.4004) (-4.4613, -2.3508) knots 0 0 0 1 1 1
  spline S63 degree 2 poles (-4.4613, -2.3508) (-4.3871, -2.3012) (-4.2822, -2.2756) knots 0 0 0 1 1 1
  spline S64 degree 2 poles (-4.2822, -2.2756) (-4.1774, -2.25) (-4.0413, -2.25) knots 0 0 0 1 1 1
  line L76 (-92.4451, -10.3) -> (-92.2609, -10.3)
  line L77 (-92.2609, -10.3) -> (-92.2609, -11.4736)
  spline S65 degree 2 poles (-92.2609, -11.4736) (-92.1944, -11.4102) (-92.0865, -11.3467) knots 0 0 0 1 1 1
  spline S66 degree 2 poles (-92.0865, -11.3467) (-91.9785, -11.2833) (-91.8926, -11.2516) knots 0 0 0 1 1 1
  line L78 (-91.8926, -11.2516) -> (-91.8926, -11.4296)
  spline S67 degree 2 poles (-91.8926, -11.4296) (-92.0471, -11.5023) (-92.1627, -11.6056) knots 0 0 0 1 1 1
  spline S68 degree 2 poles (-92.1627, -11.6056) (-92.2783, -11.7089) (-92.3264, -11.8061) knots 0 0 0 1 1 1
  line L79 (-92.3264, -11.8061) -> (-92.4451, -11.8061)
  line L80 (-92.4451, -11.8061) -> (-92.4451, -10.3)
  line L81 (-93.8847, -10.477) -> (-93.8847, -10.3)
  line L82 (-93.8847, -10.3) -> (-92.8932, -10.3)
  spline S69 degree 2 poles (-92.8932, -10.3) (-92.8912, -10.3665) (-92.9147, -10.4279) knots 0 0 0 1 1 1
  spline S70 degree 2 poles (-92.9147, -10.4279) (-92.9526, -10.5292) (-93.036, -10.6274) knots 0 0 0 1 1 1
  spline S71 degree 2 poles (-93.036, -10.6274) (-93.1194, -10.7256) (-93.2769, -10.8546) knots 0 0 0 1 1 1
  spline S72 degree 2 poles (-93.2769, -10.8546) (-93.5215, -11.0551) (-93.6074, -11.1723) knots 0 0 0 1 1 1
  spline S73 degree 2 poles (-93.6074, -11.1723) (-93.6934, -11.2894) (-93.6934, -11.3938) knots 0 0 0 1 1 1
  spline S74 degree 2 poles (-93.6934, -11.3938) (-93.6934, -11.5033) (-93.6151, -11.5785) knots 0 0 0 1 1 1
  spline S75 degree 2 poles (-93.6151, -11.5785) (-93.5368, -11.6537) (-93.411, -11.6537) knots 0 0 0 1 1 1
  spline S76 degree 2 poles (-93.411, -11.6537) (-93.278, -11.6537) (-93.1982, -11.5739) knots 0 0 0 1 1 1
  spline S77 degree 2 poles (-93.1982, -11.5739) (-93.1183, -11.4941) (-93.1173, -11.3529) knots 0 0 0 1 1 1
  line L83 (-93.1173, -11.3529) -> (-92.928, -11.3723)
  spline S78 degree 2 poles (-92.928, -11.3723) (-92.9475, -11.5841) (-93.0744, -11.6951) knots 0 0 0 1 1 1
  spline S79 degree 2 poles (-93.0744, -11.6951) (-93.2012, -11.8061) (-93.4151, -11.8061) knots 0 0 0 1 1 1
  spline S80 degree 2 poles (-93.4151, -11.8061) (-93.631, -11.8061) (-93.7568, -11.6864) knots 0 0 0 1 1 1
  spline S81 degree 2 poles (-93.7568, -11.6864) (-93.8827, -11.5667) (-93.8827, -11.3897) knots 0 0 0 1 1 1
  spline S82 degree 2 poles (-93.8827, -11.3897) (-93.8827, -11.2997) (-93.8458, -11.2127) knots 0 0 0 1 1 1
  spline S83 degree 2 poles (-93.8458, -11.2127) (-93.809, -11.1257) (-93.7236, -11.0295) knots 0 0 0 1 1 1
  spline S84 degree 2 poles (-93.7236, -11.0295) (-93.6381, -10.9334) (-93.4396, -10.7656) knots 0 0 0 1 1 1
  spline S85 degree 2 poles (-93.4396, -10.7656) (-93.2739, -10.6264) (-93.2268, -10.5768) knots 0 0 0 1 1 1
  spline S86 degree 2 poles (-93.2268, -10.5768) (-93.1797, -10.5271) (-93.149, -10.477) knots 0 0 0 1 1 1
  line L84 (-93.149, -10.477) -> (-93.8847, -10.477)
  line L85 (-94.5856, -10.3) -> (-94.0044, -11.8)
  line L86 (-94.0044, -11.8) -> (-94.2193, -11.8)
  line L87 (-94.2193, -11.8) -> (-94.6091, -10.7103)
  spline S87 degree 2 poles (-94.6091, -10.7103) (-94.6562, -10.5793) (-94.6879, -10.4647) knots 0 0 0 1 1 1
  spline S88 degree 2 poles (-94.6879, -10.4647) (-94.7227, -10.5875) (-94.7688, -10.7103) knots 0 0 0 1 1 1
  line L88 (-94.7688, -10.7103) -> (-95.1739, -11.8)
  line L89 (-95.1739, -11.8) -> (-95.3765, -11.8)
  line L90 (-95.3765, -11.8) -> (-94.7892, -10.3)
  line L91 (-94.7892, -10.3) -> (-94.5856, -10.3)
  line L92 (-95.9178, -10.5425) -> (-95.9178, -10.9538)
  line L93 (-95.9178, -10.9538) -> (-95.5095, -10.9538)
  line L94 (-95.5095, -10.9538) -> (-95.5095, -11.1257)
  line L95 (-95.5095, -11.1257) -> (-95.9178, -11.1257)
  line L96 (-95.9178, -11.1257) -> (-95.9178, -11.534)
  line L97 (-95.9178, -11.534) -> (-96.0917, -11.534)
  line L98 (-96.0917, -11.534) -> (-96.0917, -11.1257)
  line L99 (-96.0917, -11.1257) -> (-96.5, -11.1257)
  line L100 (-96.5, -11.1257) -> (-96.5, -10.9538)
  line L101 (-96.5, -10.9538) -> (-96.0917, -10.9538)
  line L102 (-96.0917, -10.9538) -> (-96.0917, -10.5425)
  line L103 (-96.0917, -10.5425) -> (-95.9178, -10.5425)
  line L104 (-93.6126, -2.3) -> (-93.6126, -3.8)
  line L105 (-93.6126, -3.8) -> (-94.1293, -3.8)
  spline S89 degree 2 poles (-94.1293, -3.8) (-94.3042, -3.8) (-94.3963, -3.7785) knots 0 0 0 1 1 1
  spline S90 degree 2 poles (-94.3963, -3.7785) (-94.5252, -3.7488) (-94.6163, -3.6711) knots 0 0 0 1 1 1
  spline S91 degree 2 poles (-94.6163, -3.6711) (-94.735, -3.5708) (-94.7938, -3.4148) knots 0 0 0 1 1 1
  spline S92 degree 2 poles (-94.7938, -3.4148) (-94.8527, -3.2587) (-94.8527, -3.0582) knots 0 0 0 1 1 1
  spline S93 degree 2 poles (-94.8527, -3.0582) (-94.8527, -2.8873) (-94.8128, -2.7553) knots 0 0 0 1 1 1
  spline S94 degree 2 poles (-94.8128, -2.7553) (-94.7729, -2.6233) (-94.7104, -2.5369) knots 0 0 0 1 1 1
  spline S95 degree 2 poles (-94.7104, -2.5369) (-94.648, -2.4504) (-94.5738, -2.4008) knots 0 0 0 1 1 1
  spline S96 degree 2 poles (-94.5738, -2.4008) (-94.4997, -2.3512) (-94.3948, -2.3256) knots 0 0 0 1 1 1
  spline S97 degree 2 poles (-94.3948, -2.3256) (-94.2899, -2.3) (-94.1538, -2.3) knots 0 0 0 1 1 1
  line L106 (-94.1538, -2.3) -> (-93.6126, -2.3)
  line L107 (-93.8111, -2.477) -> (-94.1313, -2.477)
  spline S98 degree 2 poles (-94.1313, -2.477) (-94.2797, -2.477) (-94.3641, -2.5046) knots 0 0 0 1 1 1
  spline S99 degree 2 poles (-94.3641, -2.5046) (-94.4485, -2.5323) (-94.4986, -2.5824) knots 0 0 0 1 1 1
  spline S100 degree 2 poles (-94.4986, -2.5824) (-94.5692, -2.653) (-94.6086, -2.7722) knots 0 0 0 1 1 1
  spline S101 degree 2 poles (-94.6086, -2.7722) (-94.648, -2.8914) (-94.648, -3.0613) knots 0 0 0 1 1 1
  spline S102 degree 2 poles (-94.648, -3.0613) (-94.648, -3.2966) (-94.5708, -3.423) knots 0 0 0 1 1 1
  spline S103 degree 2 poles (-94.5708, -3.423) (-94.4935, -3.5493) (-94.383, -3.5923) knots 0 0 0 1 1 1
  spline S104 degree 2 poles (-94.383, -3.5923) (-94.3032, -3.623) (-94.1262, -3.623) knots 0 0 0 1 1 1
  line L108 (-94.1262, -3.623) -> (-93.8111, -3.623)
  line L109 (-93.8111, -3.623) -> (-93.8111, -2.477)
  spline S105 degree 2 poles (-95.0655, -3.0306) (-95.0655, -3.404) (-95.266, -3.6153) knots 0 0 0 1 1 1
  spline S106 degree 2 poles (-95.266, -3.6153) (-95.4666, -3.8266) (-95.7838, -3.8266) knots 0 0 0 1 1 1
  spline S107 degree 2 poles (-95.7838, -3.8266) (-95.9915, -3.8266) (-96.1583, -3.7274) knots 0 0 0 1 1 1
  spline S108 degree 2 poles (-96.1583, -3.7274) (-96.325, -3.6281) (-96.4125, -3.4506) knots 0 0 0 1 1 1
  spline S109 degree 2 poles (-96.4125, -3.4506) (-96.5, -3.2731) (-96.5, -3.048) knots 0 0 0 1 1 1
  spline S110 degree 2 poles (-96.5, -3.048) (-96.5, -2.8198) (-96.4079, -2.6397) knots 0 0 0 1 1 1
  spline S111 degree 2 poles (-96.4079, -2.6397) (-96.3158, -2.4596) (-96.147, -2.367) knots 0 0 0 1 1 1
  spline S112 degree 2 poles (-96.147, -2.367) (-95.9782, -2.2744) (-95.7827, -2.2744) knots 0 0 0 1 1 1
  spline S113 degree 2 poles (-95.7827, -2.2744) (-95.5709, -2.2744) (-95.4042, -2.3767) knots 0 0 0 1 1 1
  spline S114 degree 2 poles (-95.4042, -2.3767) (-95.2374, -2.4791) (-95.1514, -2.6561) knots 0 0 0 1 1 1
  spline S115 degree 2 poles (-95.1514, -2.6561) (-95.0655, -2.8331) (-95.0655, -3.0306) knots 0 0 0 1 1 1
  spline S116 degree 2 poles (-95.2701, -3.0275) (-95.2701, -2.7563) (-95.4159, -2.6003) knots 0 0 0 1 1 1
  spline S117 degree 2 poles (-95.4159, -2.6003) (-95.5617, -2.4443) (-95.7817, -2.4443) knots 0 0 0 1 1 1
  spline S118 degree 2 poles (-95.7817, -2.4443) (-96.0058, -2.4443) (-96.1506, -2.6018) knots 0 0 0 1 1 1
  spline S119 degree 2 poles (-96.1506, -2.6018) (-96.2954, -2.7594) (-96.2954, -3.049) knots 0 0 0 1 1 1
  spline S120 degree 2 poles (-96.2954, -3.049) (-96.2954, -3.2321) (-96.2335, -3.3687) knots 0 0 0 1 1 1
  spline S121 degree 2 poles (-96.2335, -3.3687) (-96.1716, -3.5053) (-96.0524, -3.5805) knots 0 0 0 1 1 1
  spline S122 degree 2 poles (-96.0524, -3.5805) (-95.9332, -3.6557) (-95.7848, -3.6557) knots 0 0 0 1 1 1
  spline S123 degree 2 poles (-95.7848, -3.6557) (-95.574, -3.6557) (-95.4221, -3.5109) knots 0 0 0 1 1 1
  spline S124 degree 2 poles (-95.4221, -3.5109) (-95.2701, -3.3662) (-95.2701, -3.0275) knots 0 0 0 1 1 1
  line L110 (-92.8186, -0.8883) -> (-92.8186, -1.0643)
  line L111 (-92.8186, -1.0643) -> (-93.454, -1.0653)
  line L112 (-93.454, -1.0653) -> (-93.454, -0.5087)
  spline S125 degree 2 poles (-93.454, -0.5087) (-93.3076, -0.3921) (-93.1521, -0.3333) knots 0 0 0 1 1 1
  spline S126 degree 2 poles (-93.1521, -0.3333) (-92.9966, -0.2744) (-92.8329, -0.2744) knots 0 0 0 1 1 1
  spline S127 degree 2 poles (-92.8329, -0.2744) (-92.6119, -0.2744) (-92.4313, -0.3691) knots 0 0 0 1 1 1
  spline S128 degree 2 poles (-92.4313, -0.3691) (-92.2507, -0.4637) (-92.1586, -0.6428) knots 0 0 0 1 1 1
  spline S129 degree 2 poles (-92.1586, -0.6428) (-92.0665, -0.8218) (-92.0665, -1.0428) knots 0 0 0 1 1 1
  spline S130 degree 2 poles (-92.0665, -1.0428) (-92.0665, -1.2618) (-92.1581, -1.4516) knots 0 0 0 1 1 1
  spline S131 degree 2 poles (-92.1581, -1.4516) (-92.2497, -1.6414) (-92.4216, -1.7335) knots 0 0 0 1 1 1
  spline S132 degree 2 poles (-92.4216, -1.7335) (-92.5935, -1.8256) (-92.8175, -1.8256) knots 0 0 0 1 1 1
  spline S133 degree 2 poles (-92.8175, -1.8256) (-92.9802, -1.8256) (-93.1117, -1.7729) knots 0 0 0 1 1 1
  spline S134 degree 2 poles (-93.1117, -1.7729) (-93.2432, -1.7202) (-93.3179, -1.6261) knots 0 0 0 1 1 1
  spline S135 degree 2 poles (-93.3179, -1.6261) (-93.3926, -1.5319) (-93.4314, -1.3805) knots 0 0 0 1 1 1
  line L113 (-93.4314, -1.3805) -> (-93.2524, -1.3314)
  spline S136 degree 2 poles (-93.2524, -1.3314) (-93.2186, -1.446) (-93.1685, -1.5115) knots 0 0 0 1 1 1
  spline S137 degree 2 poles (-93.1685, -1.5115) (-93.1183, -1.5769) (-93.0252, -1.6163) knots 0 0 0 1 1 1
  spline S138 degree 2 poles (-93.0252, -1.6163) (-92.9321, -1.6557) (-92.8186, -1.6557) knots 0 0 0 1 1 1
  spline S139 degree 2 poles (-92.8186, -1.6557) (-92.6825, -1.6557) (-92.5832, -1.6143) knots 0 0 0 1 1 1
  spline S140 degree 2 poles (-92.5832, -1.6143) (-92.484, -1.5729) (-92.4231, -1.5053) knots 0 0 0 1 1 1
  spline S141 degree 2 poles (-92.4231, -1.5053) (-92.3622, -1.4378) (-92.3284, -1.357) knots 0 0 0 1 1 1
  spline S142 degree 2 poles (-92.3284, -1.357) (-92.2711, -1.2178) (-92.2711, -1.0551) knots 0 0 0 1 1 1
  spline S143 degree 2 poles (-92.2711, -1.0551) (-92.2711, -0.8546) (-92.3402, -0.7195) knots 0 0 0 1 1 1
  spline S144 degree 2 poles (-92.3402, -0.7195) (-92.4093, -0.5844) (-92.5413, -0.519) knots 0 0 0 1 1 1
  spline S145 degree 2 poles (-92.5413, -0.519) (-92.6733, -0.4535) (-92.8216, -0.4535) knots 0 0 0 1 1 1
  spline S146 degree 2 poles (-92.8216, -0.4535) (-92.9505, -0.4535) (-93.0733, -0.5031) knots 0 0 0 1 1 1
  spline S147 degree 2 poles (-93.0733, -0.5031) (-93.1961, -0.5527) (-93.2595, -0.609) knots 0 0 0 1 1 1
  line L114 (-93.2595, -0.609) -> (-93.2595, -0.8883)
  line L115 (-93.2595, -0.8883) -> (-92.8186, -0.8883)
  line L116 (-93.7445, -0.3) -> (-93.7445, -1.8)
  line L117 (-93.7445, -1.8) -> (-93.9482, -1.8)
  line L118 (-93.9482, -1.8) -> (-94.736, -0.6223)
  line L119 (-94.736, -0.6223) -> (-94.736, -1.8)
  line L120 (-94.736, -1.8) -> (-94.9263, -1.8)
  line L121 (-94.9263, -1.8) -> (-94.9263, -0.3)
  line L122 (-94.9263, -0.3) -> (-94.7227, -0.3)
  line L123 (-94.7227, -0.3) -> (-93.9349, -1.4787)
  line L124 (-93.9349, -1.4787) -> (-93.9349, -0.3)
  line L125 (-93.9349, -0.3) -> (-93.7445, -0.3)
  line L126 (-95.2599, -0.3) -> (-95.2599, -1.8)
  line L127 (-95.2599, -1.8) -> (-95.7766, -1.8)
  spline S148 degree 2 poles (-95.7766, -1.8) (-95.9516, -1.8) (-96.0437, -1.7785) knots 0 0 0 1 1 1
  spline S149 degree 2 poles (-96.0437, -1.7785) (-96.1726, -1.7488) (-96.2636, -1.6711) knots 0 0 0 1 1 1
  spline S150 degree 2 poles (-96.2636, -1.6711) (-96.3823, -1.5708) (-96.4412, -1.4148) knots 0 0 0 1 1 1
  spline S151 degree 2 poles (-96.4412, -1.4148) (-96.5, -1.2587) (-96.5, -1.0582) knots 0 0 0 1 1 1
  spline S152 degree 2 poles (-96.5, -1.0582) (-96.5, -0.8873) (-96.4601, -0.7553) knots 0 0 0 1 1 1
  spline S153 degree 2 poles (-96.4601, -0.7553) (-96.4202, -0.6233) (-96.3578, -0.5369) knots 0 0 0 1 1 1
  spline S154 degree 2 poles (-96.3578, -0.5369) (-96.2954, -0.4504) (-96.2212, -0.4008) knots 0 0 0 1 1 1
  spline S155 degree 2 poles (-96.2212, -0.4008) (-96.147, -0.3512) (-96.0421, -0.3256) knots 0 0 0 1 1 1
  spline S156 degree 2 poles (-96.0421, -0.3256) (-95.9372, -0.3) (-95.8012, -0.3) knots 0 0 0 1 1 1
  line L128 (-95.8012, -0.3) -> (-95.2599, -0.3)
  line L129 (-95.4584, -0.477) -> (-95.7786, -0.477)
  spline S157 degree 2 poles (-95.7786, -0.477) (-95.927, -0.477) (-96.0114, -0.5046) knots 0 0 0 1 1 1
  spline S158 degree 2 poles (-96.0114, -0.5046) (-96.0958, -0.5323) (-96.146, -0.5824) knots 0 0 0 1 1 1
  spline S159 degree 2 poles (-96.146, -0.5824) (-96.2166, -0.653) (-96.256, -0.7722) knots 0 0 0 1 1 1
  spline S160 degree 2 poles (-96.256, -0.7722) (-96.2954, -0.8914) (-96.2954, -1.0613) knots 0 0 0 1 1 1
  spline S161 degree 2 poles (-96.2954, -1.0613) (-96.2954, -1.2966) (-96.2181, -1.423) knots 0 0 0 1 1 1
  spline S162 degree 2 poles (-96.2181, -1.423) (-96.1409, -1.5493) (-96.0304, -1.5923) knots 0 0 0 1 1 1
  spline S163 degree 2 poles (-96.0304, -1.5923) (-95.9505, -1.623) (-95.7735, -1.623) knots 0 0 0 1 1 1
  line L130 (-95.7735, -1.623) -> (-95.4584, -1.623)
  line L131 (-95.4584, -1.623) -> (-95.4584, -0.477)
extrude "Extrusion5" add sketch "Skizze4" along normal blind 0.01 contours L76 L77 S65 S66 L78 S67 S68 L79 L80 | L81 L82 S69 S70 S71 S72 S73 S74 S75 S76 S77 L83 S78 S79 S80 S81 S82 S83 S84 S85 S86 L84 | L85 L86 L87 S87 S88 L88 L89 L90 L91 | L92 L93 L94 L95 L96 L97 L98 L99 L100 L101 L102 L103 | L104 L105 S89 S90 S91 S92 S93 S94 S95 S96 S97 L106 | S105 S106 S107 S108 S109 S110 S111 S112 S113 S114 S115 | L110 L111 L112 S125 S126 S127 S128 S129 S130 S131 S132 S133 S134 S135 L113 S136 S137 S138 S139 S140 S141 S142 S143 S144 S145 S146 S147 L114 L115 | L116 L117 L118 L119 L120 L121 L122 L123 L124 L125 | L126 L127 S148 S149 S150 S151 S152 S153 S154 S155 S156 L128 bodies 1
equation "d6 = 0deg 0'"
equation "d8 = 0deg 0'"
equation "d16 = 0deg 0'"
equation "d35 = 0deg 0'"
equation "d44 = 0deg 0'"

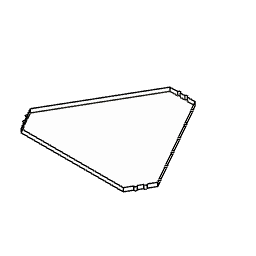
design "Light_Guide_Panel"
Autodesk Fusion 360 part; units mm, degrees
sketch "Skizze1" plane through (0, 0, 0) normal (0, 0, 1) x (1, 0, 0)
  line L0 (-56.2917, 0) -> (56.2917, 0)
  line L1 (56.2917, 0) -> (70.1481, 24)
  line L2 (70.1481, 24) -> (13.8564, 121.5)
  line L3 (13.8564, 121.5) -> (-13.8564, 121.5)
  line L4 (-13.8564, 121.5) -> (-70.1481, 24)
  line L5 (-70.1481, 24) -> (-56.2917, 0)
  line L6 (0, 0) -> (0, 121.5)
  line L7 (-63.2199, 12) -> (42.0022, 72.75)
  line L8 (63.2199, 12) -> (-42.0022, 72.75)
  circle A0 centre (-4, 121.5) radius 1.4
  circle A1 centre (4, 121.5) radius 1.4
  circle A2 centre (-61.2199, 8.5359) radius 1.4
  circle A3 centre (-65.2199, 15.4641) radius 1.4
  circle A4 centre (65.2199, 15.4641) radius 1.4
  circle A5 centre (61.2199, 8.5359) radius 1.4
  point P0 (0, 48.5)
  dimension "d1" = 48.5
  dimension "d2" = 73
  dimension "d3" = 27.7128
  dimension "d4" = 112.5833
  dimension "d18" = 2.8
  dimension "d19" = 8
  dimension "d21" = 360
  constraint horizontal L0
  constraint parallel L0 L3
  constraint parallel L1 L4
  constraint equal L1 L3
  constraint equal L1 L5
  constraint equal L2 L4
  constraint equal L0 L2
  constraint coincident L6.start L0
  constraint coincident L6.start origin
  constraint coincident L3 L6.end
  constraint perpendicular L3 L6
  constraint symmetric L2 L4 L6
  constraint symmetric L1 L5 L6
  constraint midpoint L5 L7.start
  constraint midpoint L2 L7.end
  constraint midpoint L1 L8.start
  constraint midpoint L4 L8.end
  constraint coincident L7 P0
  constraint coincident L6 P0
  constraint coincident L3 A0.centre
  constraint symmetric L6 A0 A1
  measures "d1" distance of L0 P0
  measures "d2" distance of L3 P0
  measures "d3" distance of L2.end L3.end
  measures "d4" distance of L0.start L0.end
  measures "d18" diameter of A0
  measures "d19" distance of A0.centre A1.centre
extrude "Extrusion1" add sketch "Skizze1" along normal blind 4
sketch "Skizze2" plane through (0, 0, 4) normal (0, 0, 1) x (-1, 0, 0)
  arc A0 (-60.5199, -7.3235) -> (-61.9199, -9.7483) centre (-61.2199, -8.5359) ccw
  line L0 (-61.9199, -9.7483) -> (-64.5199, -14.2517)
  arc A1 (-64.5199, -14.2517) -> (-65.9199, -16.6765) centre (-65.2199, -15.4641) ccw
  line L1 (-65.9199, -16.6765) -> (-70.1481, -24)
  line L2 (-70.1481, -24) -> (-13.8564, -121.5)
  line L3 (-13.8564, -121.5) -> (-5.4, -121.5)
  arc A2 (-5.4, -121.5) -> (-2.6, -121.5) centre (-4, -121.5) ccw
  line L4 (-2.6, -121.5) -> (2.6, -121.5)
  arc A3 (2.6, -121.5) -> (5.4, -121.5) centre (4, -121.5) ccw
  line L5 (5.4, -121.5) -> (13.8564, -121.5)
  line L6 (13.8564, -121.5) -> (70.1481, -24)
  line L7 (70.1481, -24) -> (65.9199, -16.6765)
  arc A4 (65.9199, -16.6765) -> (64.5199, -14.2517) centre (65.2199, -15.4641) ccw
  line L8 (64.5199, -14.2517) -> (61.9199, -9.7483)
  arc A5 (61.9199, -9.7483) -> (60.5199, -7.3235) centre (61.2199, -8.5359) ccw
  line L9 (60.5199, -7.3235) -> (56.2917, 0)
  line L10 (56.2917, 0) -> (-56.2917, 0)
  line L11 (-56.2917, 0) -> (-60.5199, -7.3235)
equation "d6 = 0deg 0'"
equation "d10 = 0deg 0'"
equation "d21 = 360deg 0'"

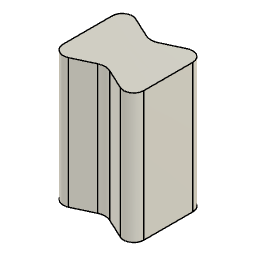
design "Verbinder"
Autodesk Fusion 360 part; units mm, degrees
sketch "Skizze1" plane through (0, 0, 0) normal (0, 0, 1) x (1, 0, 0)
  line L0 (0, 1.4943) -> (2.8, 2.8)
  line L1 (2.8, 2.8) -> (2.8, -2.8)
  line L2 (2.8, -2.8) -> (0, -1.4943)
  line L3 (0, -1.4943) -> (0, 1.4943)
  line L4 (2.8, 0) -> (0, 0)
  line L5 (0, 1.4943) -> (-2.8, 2.8)
  line L6 (-2.8, 2.8) -> (-2.8, -2.8)
  line L7 (-2.8, -2.8) -> (0, -1.4943)
  dimension "d1" = 5.6
  dimension "d2" = 5.6
  dimension "d3" = 50
  constraint vertical L1
  constraint vertical L3
  constraint midpoint L1 L4.start
  constraint coincident L4.end origin
  constraint perpendicular L3 L4
  constraint symmetric L0 L2 L4
  constraint symmetric L0.start L3 L5.start
  constraint symmetric L0.end L3 L5.end
  constraint symmetric L1.end L3 L6.end
  constraint symmetric L2.end L3 L7.end
  constraint coincident L4.end L3
  measures "d1" distance of L1 L6
  measures "d2" distance of L0.end L1.end
  measures "d3" angle of L0 L2
extrude "Extrusion1" add sketch "Skizze1" along normal blind 9
fillet "Abrundung1" radius 0.7 4 edges at (-2.8, -2.8, 4.5) (2.8, -2.8, 4.5) (2.8, 2.8, 4.5) (-2.8, 2.8, 4.5)
fillet "Abrundung2" radius 1 2 edges at (0, -1.4943, 4.5) (0, 1.4943, 4.5)
equation "d5 = 0deg 0'"

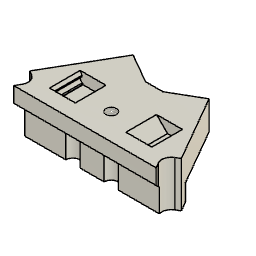
design "Deckel_mitte"
Autodesk Fusion 360 part; units mm, degrees
sketch "Skizze1" plane through (0, 0, 0) normal (0, 0, 1) x (1, 0, 0)
  line L0 (-17.5, 0) -> (-7.95, 16.5411)
  line L1 (7.95, 16.5411) -> (17.5, 0)
  line L2 (17.5, 0) -> (-17.5, 0)
  line L3 (0, 0) -> (0, 24.5)
  line L4 (-14.7, 4.8497) -> (-7.512, 0.6997)
  line L5 (-7.512, 0.6997) -> (-0.762, 12.3911)
  line L6 (-0.762, 12.3911) -> (-7.95, 16.5411)
  line L7 (-17.5, 0) -> (-18.366, -1.5)
  line L8 (17.5, 0) -> (18.366, -1.5)
  line L9 (-18.366, -1.5) -> (18.366, -1.5)
  line L10 (-1.8167, 13) -> (1.8167, 13)
  line L11 (0.762, 12.3911) -> (7.95, 16.5411)
  line L12 (7.512, 0.6997) -> (0.762, 12.3911)
  line L13 (14.7, 4.8497) -> (7.512, 0.6997)
  point P0 (0, 4)
  dimension "d1" = 60
  dimension "d10" = 4
  dimension "d28" = 35
  dimension "d31" = 13.5
  dimension "d32" = 5.6
  dimension "d33" = 8.3
  dimension "d57" = 1.5
  dimension "d79" = 13
  constraint midpoint L2 L3.start
  constraint vertical L3
  constraint coincident L3.start origin
  constraint coincident L3 P0
  constraint coincident L0 L4.start
  constraint perpendicular L5 L6
  constraint parallel L0 L5
  constraint parallel L4 L6
  constraint coincident L7.end L9.start
  constraint collinear L0 L7
  constraint collinear L1 L8
  constraint horizontal L9
  constraint coincident L8.end L9.end
  constraint coincident L6 L10.start
  constraint symmetric L3 L4.start L13.start
  constraint symmetric L3 L4.end L12.start
  constraint symmetric L3 L5.end L11.start
  constraint symmetric L3 L0.end L1.start
  constraint coincident L11 L10.end
  constraint horizontal L10
  measures "d1" angle of L0 L1
  measures "d10" distance of L2 P0
  measures "d28" distance of L0.start L1.end
  measures "d31" distance of L4 L6
  measures "d32" distance of L0.start L4
  measures "d33" distance of L4.start L4.end
  measures "d57" distance of L2 L9
  measures "d79" distance of L3.start L10
extrude "Extrusion1" add sketch "Skizze1" along normal blind 9.5 contours L0 L2 L3 L4 L5 L6 L10 | L0 L4 L5 L6 | L1 L2 L3 L10 L11 L12 L13 | L1 L11 L12 L13